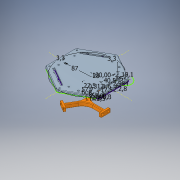
# Autodesk Inventor part: Stewart-Platform-Base-Innen
Saved by Autodesk Inventor 2018.2 (Build 222227000, 227)
## iProperties
Created: 2018-02-17
Part Number: Stewart-Platform-Base-Innen
Material: Generisch
Document SubType Name: Modeling
Designer: JochenAlt
Density: 1 g/cm^3
Appearance: Vorgabe
Author: JochenAlt
Autodesk Inventor part; units mm, degrees
ref_plane "YZ Plane" through (0, 0, 0) normal (1, 0, 0) x (0, 1, 0)
ref_plane "XZ Plane" through (0, 0, 0) normal (0, 1, 0) x (-1, 0, 0)
sketch "Skizze1" plane through (0, 0, 0) normal (0, 0, 1) x (1, 0, 0)
  line L0 (0, 78.1556) -> (0, -78.0893) construction
  line L1 (-71.7181, 0) -> (82.4088, 0) construction
  line L2 (31.6, 28.85) -> (44.1, 28.85) construction
  line L3 (47.4, 25.55) -> (47.4, -25.55) construction
  line L4 (44.1, -28.85) -> (31.6, -28.85) construction
  line L5 (28.3, -25.55) -> (28.3, 25.55) construction
  arc A0 (31.6, 28.85) -> (28.3, 25.55) centre (31.6, 25.55) ccw construction
  arc A1 (47.4, 25.55) -> (44.1, 28.85) centre (44.1, 25.55) ccw construction
  arc A2 (44.1, -28.85) -> (47.4, -25.55) centre (44.1, -25.55) ccw construction
  arc A3 (28.3, -25.55) -> (31.6, -28.85) centre (31.6, -25.55) ccw construction
  circle A4 centre (31.6, 25.55) radius 1.25
  circle A5 centre (44.1, 25.55) radius 1.25
  circle A6 centre (31.6, -25.55) radius 1.25
  circle A7 centre (44.1, -25.55) radius 1.25
  line L6 (41.4, 20.25) -> (41.4, -20.25)
  line L7 (38.3, 20.25) -> (38.3, -20.25)
  line L8 (38.3, 20.25) -> (41.4, 20.25)
  line L9 (38.3, -20.25) -> (41.4, -20.25)
  line L10 (38.3, 0.8) -> (41.4, 0.8)
  line L11 (38.3, -0.8) -> (41.4, -0.8)
  line L12 (41.4, 11.55) -> (44.416, 11.55)
  line L13 (44.416, 11.55) -> (44.416, 8.75)
  line L14 (44.416, 8.75) -> (41.4, 8.75)
  line L15 (41.4, -8.75) -> (44.416, -8.75)
  line L16 (44.416, -8.75) -> (44.416, -11.55)
  line L17 (44.416, -11.55) -> (41.4, -11.55)
  line L18 (44.1, 29.15) -> (31.6, 29.15)
  arc A8 (31.6, 29.15) -> (28, 25.55) centre (31.6, 25.55) ccw
  line L19 (28, 25.55) -> (28, -25.55)
  arc A9 (28, -25.55) -> (31.6, -29.15) centre (31.6, -25.55) ccw
  line L20 (31.6, -29.15) -> (44.1, -29.15)
  arc A10 (44.1, -29.15) -> (47.7, -25.55) centre (44.1, -25.55) ccw
  line L21 (47.7, -25.55) -> (47.7, 25.55)
  arc A11 (47.7, 25.55) -> (44.1, 29.15) centre (44.1, 25.55) ccw
  line L22 (26.117, -29.2238) -> (28.6093, -27.5539) construction
  line L23 (49.7, 0) -> (47.7, 0) construction
  circle A12 centre (0, 0) radius 49.7 construction
  line L24 (35.8007, 29.2532) -> (34.3005, 27.9307) construction
  line L25 (47.7, -19.95) -> (41.4, -19.95)
  line L26 (47.7, 19.95) -> (41.4, 19.95)
  arc A13 (3.1946, 52.7667) -> (-1.7231, 54.0844) centre (0.0769, 50.9667) ccw
  circle A14 centre (0.0769, 50.9667) radius 1.25
  line L27 (-1.7231, 54.0844) -> (-45.9769, 28.5344)
  line L28 (-6.5728, 51.2844) -> (-3.4228, 45.8285)
  line L29 (-12.2054, 44.2404) -> (-10.6974, 41.6285)
  line L30 (-14.6303, 42.8404) -> (-12.2054, 44.2404)
  line L31 (-13.1223, 40.2285) -> (-14.6303, 42.8404)
  line L32 (-38.237, 25.7285) -> (-3.163, 45.9785)
  line L33 (-1.613, 43.2938) -> (-3.163, 45.9785)
  line L34 (-36.687, 23.0438) -> (-1.613, 43.2938)
  line L35 (-18.4572, 33.5688) -> (-20.0072, 36.2535)
  line L36 (-19.8428, 32.7688) -> (-21.3928, 35.4535)
  line L37 (-32.2106, 32.6904) -> (-29.7857, 34.0904)
  line L38 (-29.7857, 34.0904) -> (-28.2777, 31.4785)
  line L39 (-30.7026, 30.0785) -> (-32.2106, 32.6904)
  line L40 (-41.1272, 31.3344) -> (-37.9772, 25.8785)
  line L41 (-36.687, 23.0438) -> (-38.237, 25.7285)
  arc A15 (-45.9769, 28.5344) -> (-47.2946, 23.6167) centre (-44.1769, 25.4167) ccw
  circle A16 centre (-44.1769, 25.4167) radius 1.25
  line L42 (-47.2946, 23.6167) -> (-41.0446, 12.7914)
  circle A17 centre (6.3269, 40.1414) radius 1.25
  arc A18 (8.1269, 37.0237) -> (9.4446, 41.9414) centre (6.3269, 40.1414) ccw
  line L43 (-36.1269, 11.4737) -> (8.1269, 37.0237)
  circle A19 centre (-37.9269, 14.5914) radius 1.25
  arc A20 (-41.0446, 12.7914) -> (-36.1269, 11.4737) centre (-37.9269, 14.5914) ccw
  line L44 (9.4446, 41.9414) -> (3.1946, 52.7667)
  arc A21 (-47.2946, -23.6167) -> (-45.9769, -28.5344) centre (-44.1769, -25.4167) ccw
  circle A22 centre (-44.1769, -25.4167) radius 1.25
  line L45 (-45.9769, -28.5344) -> (-1.7231, -54.0844)
  line L46 (-41.1272, -31.3344) -> (-37.9772, -25.8785)
  line L47 (-32.2106, -32.6904) -> (-30.7026, -30.0785)
  line L48 (-29.7857, -34.0904) -> (-32.2106, -32.6904)
  line L49 (-28.2777, -31.4785) -> (-29.7857, -34.0904)
  line L50 (-3.163, -45.9785) -> (-38.237, -25.7285)
  line L51 (-36.687, -23.0438) -> (-38.237, -25.7285)
  line L52 (-1.613, -43.2938) -> (-36.687, -23.0438)
  line L53 (-19.8428, -32.7688) -> (-21.3928, -35.4535)
  line L54 (-18.4572, -33.5688) -> (-20.0072, -36.2535)
  line L55 (-12.2054, -44.2404) -> (-14.6303, -42.8404)
  line L56 (-14.6303, -42.8404) -> (-13.1223, -40.2285)
  line L57 (-10.6974, -41.6285) -> (-12.2054, -44.2404)
  line L58 (-6.5728, -51.2844) -> (-3.4228, -45.8285)
  line L59 (-1.613, -43.2938) -> (-3.163, -45.9785)
  arc A23 (-1.7231, -54.0844) -> (3.1946, -52.7667) centre (0.0769, -50.9667) ccw
  circle A24 centre (0.0769, -50.9667) radius 1.25
  line L60 (3.1946, -52.7667) -> (9.4446, -41.9414)
  circle A25 centre (-37.9269, -14.5914) radius 1.25
  arc A26 (-36.1269, -11.4737) -> (-41.0446, -12.7914) centre (-37.9269, -14.5914) ccw
  line L61 (8.1269, -37.0237) -> (-36.1269, -11.4737)
  circle A27 centre (6.3269, -40.1414) radius 1.25
  arc A28 (9.4446, -41.9414) -> (8.1269, -37.0237) centre (6.3269, -40.1414) ccw
  line L62 (-41.0446, -12.7914) -> (-47.2946, -23.6167)
  line L63 (48.4856, -28.1531) -> (47.1957, -27.3875) construction
  line L64 (49.2, -25.55) -> (49.2, 25.55)
  line L65 (-2.3204, -55.1191) -> (-46.5743, -29.5691)
  line L66 (-46.6082, 29.6278) -> (-2.3543, 55.1778)
  arc A29 (-46.6082, 29.6278) -> (-49.0395, 25.4102) centre (-44.1769, 25.4167) ccw
  line L67 (2.4885, 55.1891) -> (46.6293, 29.9786)
  line L68 (-48.9717, -25.4231) -> (-49.0395, 25.4102)
  arc A30 (2.4885, 55.1891) -> (-2.3543, 55.1778) centre (0.0769, 50.9667) ccw
  arc A31 (49.2, 25.55) -> (46.6293, 29.9786) centre (44.1, 25.55) ccw
  arc A32 (32.9365, 29.15) -> (44.8907, 37.253) centre (44.1, 25.55) ccw
  arc A33 (46.6234, -29.982) -> (49.2, -25.55) centre (44.1, -25.55) ccw
  line L69 (46.6234, -29.982) -> (2.4494, -55.1334)
  arc A34 (-2.3204, -55.1191) -> (2.4494, -55.1334) centre (0.0769, -50.9667) ccw
  arc A35 (-48.9717, -25.4231) -> (-46.5743, -29.5691) centre (-44.1769, -25.4167) ccw
  circle A36 centre (0, 0) radius 43.5 construction
  circle A37 centre (-43.5, 0) radius 1.65
  circle A38 centre (21.75, -37.6721) radius 1.65
  circle A39 centre (21.75, 37.6721) radius 1.65
  line L70 (21.75, -37.6721) -> (0, 0) construction
  line L71 (0, 0) -> (21.75, 37.6721) construction
  line L72 (34.4282, 0) -> (34.4282, -12) construction
  line L73 (34.4282, -12) -> (6.9282, -12) construction
  point P0 (44.416, -10.15)
  point P1 (0, 0)
  point P2 (47.7, -21.4)
  point P3 (47.7, 21.4)
  point P4 (-23.85, 41.3094)
  point P5 (-5.3171, 52.0094)
  point P6 (-42.3829, 30.6094)
  point P7 (-13.4178, 43.5404)
  point P8 (9.5577, 38.5533)
  point P9 (-41.3389, 15.7397)
  point P10 (-23.85, -41.3094)
  point P11 (-42.3829, -30.6094)
  point P12 (-5.3171, -52.0094)
  point P13 (-30.9982, -33.3904)
  point P14 (-38.167, -10.9994)
  point P15 (7.0384, -43.6704)
  dimension "d1" = 57.7
  dimension "d2" = 19.1
  dimension "d3" = 3.3
  dimension "d5" = 2.5
  dimension "d6" = 6
  dimension "d7" = 3.1
  dimension "d9" = 1.6
  dimension "d10" = 2.984
  dimension "d11" = 2.8
  dimension "d12" = 17.5
  dimension "d21" = 0.3
  dimension "d22" = 3
  dimension "d34" = 2
  dimension "d35" = 2
  dimension "d105" = 360
  dimension "d107" = 40.5
  dimension "d108" = 0.3
  dimension "d140" = 1.5
  dimension "d141" = 28
  dimension "d145" = 1.5
  dimension "d148" = 87
  dimension "d149" = 3.3
  dimension "d150" = 120
  dimension "d151" = 12
  dimension "d152" = 27.5
  constraints: 138 end point, 56 point on circle, 39 centre point, 28 point on line, 22 coincident, 20 tangent, 11 horizontal, 8 equal radius, 7 parallel, 5 perpendicular, 3 line through centre, 2 midpoint, 2 vertical, 1 collinear, 1 horizontal alignment, 1 symmetric about line, 253 other
  measures "d1" distance between parallel lines of L4 L2
  measures "d2" distance between parallel lines of L3 L5
  measures "d3" radius of A0
  measures "d5" diameter of A4
  measures "d9" distance between parallel lines of L11 L10
  measures "d10" distance between parallel lines of L3 L13
  measures "d11" distance between parallel lines of L14 L12
  measures "d12" distance between parallel lines of L15 L14
  measures "d21" distance between parallel lines of L19 L5
  measures "d22" distance of L22.end L22.start
  measures "d34" distance of L23.start L23.end
  measures "d35" distance of L24.start L24.end
  measures "d107" distance between parallel lines of L8 L9
  measures "d108" distance between parallel lines of L25 L9
  measures "d140" distance of L63.start L63.end
  measures "d141" distance between parallel lines of L0 L19
  measures "d145" distance between parallel lines of L21 L64
  measures "d148" diameter of A36
  measures "d149" diameter of A37
  measures "d150" angle of L71 L70
  measures "d151" distance of L72.start L72.end
  measures "d152" distance of L72.end L73.end
extrude "Extrusion5" add sketch "Skizze1" along normal blind 4 contours A4 A32 L18 A11 L21 L26 L6 L8 L7 | A4 A32 L7 L9 L6 L25 L21 A10 L20 A9 L19 A8 L18 | A32 L21 L25 L6 L17 L16 L15 L14 L13 L12 | L6 L26 L21 A32 | L44 A18 L43 A20 L42 A15 L27 L40 L32 L41 L34 L33 L28 A13 | L28 L32 L29 L30 L31 L38 L37 L39 L40 L27 | L62 A26 L61 A28 L60 A23 L45 L58 L50 L59 L52 L51 L46 A21 | L46 L50 L47 L48 L49 L56 L55 L57 L58 L45 | A33 L69 A34 L65 A35 L68 A29 L66 A30 L67 A31 L64
extrude "Extrusion4" cut sketch "Skizze1" along normal blind 2 contours A4 A32 L18 A11 L21 L26 L6 L8 L7 | A4 A32 L7 L9 L6 L25 L21 A10 L20 A9 L19 A8 L18 | L12 L13 L14 L6 | L15 L16 L17 L6 | L44 A18 L43 A20 L42 A15 L27 L40 L32 L41 L34 L33 L28 A13 | L62 A26 L61 A28 L60 A23 L45 L58 L50 L59 L52 L51 L46 A21
ref_plane "Arbeitsebene2" through (0, 0, -40.8) normal (0, 0, 1) x (1, 0, 0)
sketch "Skizze6" plane through (0, 0, -40.8) normal (0, 0, 1) x (1, 0, 0)
  line L0 (41.4, -11.55) -> (41.4, -20.25) construction
  line L1 (41.4, -20.25) -> (38.3, -20.25) construction
  line L2 (38.3, -20.25) -> (38.3, 20.25) construction
  line L3 (41.4, 20.25) -> (41.4, 11.55) construction
  line L4 (38.3, 20.25) -> (41.4, 20.25) construction
  circle A0 centre (44.1, -25.55) radius 1.25 construction
  circle A1 centre (31.6, -25.55) radius 1.25 construction
  circle A2 centre (44.1, 25.55) radius 1.25 construction
  circle A3 centre (31.6, 25.55) radius 1.25 construction
  line L5 (34.1, 8.75) -> (34.1, -8.75)
  line L6 (34.1, 8.75) -> (31.1, 8.75)
  line L7 (41.4, -8.75) -> (41.4, 8.75) projected
  line L8 (-65.8313, 0) -> (60.3802, 0) construction
  line L9 (0, 37.52) -> (0, -37.52) construction
  line L10 (31.1, -8.75) -> (31.1, -2)
  line L11 (31.1, 2) -> (31.1, 8.75)
  line L12 (0, 0) -> (8.9019, 15.4186) construction
  line L13 (0, 0) -> (9.1171, -15.7912) construction
  arc A4 (2.7017, 4.6795) -> (12.7017, 2) centre (12.7017, 22) ccw
  arc A5 (12.7017, -2) -> (2.7017, -4.6795) centre (12.7017, -22) ccw
  line L14 (2.7017, 4.6795) -> (0, 6.2393)
  line L15 (2.7017, -4.6795) -> (0, -6.2393)
  line L16 (31.1, 2) -> (12.7017, 2)
  line L17 (31.1, -2) -> (12.7017, -2)
  line L18 (31.1, 8.75) -> (34.1, 8.75) projected
  line L19 (34.1, -8.75) -> (31.1, -8.75)
  arc A6 (0, -1.65) -> (0, 1.65) centre (0, 0) ccw
  line L20 (0, 6.2393) -> (0, 1.65)
  line L21 (0, -1.65) -> (0, -6.2393)
  line L22 (41.4, 8.75) -> (41.4, -8.75) projected
  line L23 (41.4, -8.75) -> (44.416, -8.75) projected
  line L24 (44.416, -8.75) -> (44.416, -11.55) projected
  line L25 (44.416, -11.55) -> (41.4, -11.55) projected
  line L26 (41.4, 11.55) -> (44.416, 11.55) projected
  line L27 (44.416, 11.55) -> (44.416, 8.75) projected
  line L28 (44.416, 8.75) -> (41.4, 8.75) projected
  point P0 (-47.8011, -0.8)
  dimension "d73" = 120
  dimension "d89" = 20
  dimension "d90" = 4
  dimension "d91" = 3.3
  dimension "d146" = 3
  dimension "d147" = 4.2
  constraints: 26 end point, 6 point on circle, 4 perpendicular, 4 point on line, 4 tangent, 3 centre point, 2 parallel, 1 coincident, 1 collinear, 1 other
  measures "d73" angle of L13 L12
  measures "d89" radius of A5
  measures "d90" distance between parallel lines of L16 L17
  measures "d91" diameter of A6
  measures "d146" distance between parallel lines of L11 L5
  measures "d147" distance between parallel lines of L5 L2
extrude "Extrusion9" add sketch "Skizze6" against normal blind 7.1 separate body
sketch "Skizze7" plane through (34.1, 8.75, -40.8) normal (1, 0, 0) x (0, 0, -1)
  circle A0 centre (3.8, -3.7) radius 1.7
  circle A1 centre (3.8, -13.8) radius 1.7
  line L0 (0, -17.5) -> (0, 0) construction
  line L1 (0, -8.75) -> (7.1, -8.75) construction
  line L2 (7.1, 0) -> (7.1, -17.5) construction
  point P0 (-40.8, -8.75)
  dimension "d76" = 3.4
  dimension "d77" = 10.1
  dimension "d88" = 3.3
  constraints: 2 centre point, 2 end point, 2 midpoint, 1 equal radius, 1 symmetric about line
  measures "d76" diameter of A1
  measures "d77" distance of A0.centre A1.centre
  measures "d88" distance from line of A0.centre L2
extrude "Extrusion10" cut sketch "Skizze7" against normal blind 10 bodies 1 2
pattern_circular "Runde Anordnung5" count 3 over 360 about axis through (0, 0, -10) along (0, 0, 1) of "Extrusion10", "Extrusion9" bodies 2
fillet "Rundung1" radius 1 30 edges at (2.7017, 4.6795, -40.8) (21.9009, 2, -40.8) (-9.2184, 19.9667, -40.8) (2.7017, -4.6795, -40.8) (-9.2184, -19.9667, -40.8) (21.9009, -2, -40.8) (-12.6825, -17.9667, -40.8) (-12.6825, 17.9667, -40.8) (-5.4034, 0, -40.8) (2.7017, 4.6795, -47.9) (21.9009, 2, -47.9) (-9.2184, 19.9667, -47.9) (-12.6825, 17.9667, -47.9) (-12.6825, -17.9667, -47.9) (-5.4034, 0, -47.9) (32.6, -8.75, -47.9) (32.6, 8.75, -47.9) (-8.7223, -32.6074, -47.9) (-23.8777, -23.8574, -47.9) (-23.8777, -23.8574, -40.8) (-8.7223, -32.6074, -40.8) (32.6, -8.75, -40.8) (32.6, 8.75, -40.8) (-8.7223, 32.6074, -40.8) (-8.7223, 32.6074, -47.9) (-23.8777, 23.8574, -40.8) (-23.8777, 23.8574, -47.9) (-9.2184, -19.9667, -47.9) (21.9009, -2, -47.9) (2.7017, -4.6795, -47.9)
fillet "Rundung2" radius 1 15 edges at (-24.4474, -42.3441, 4) (49.2, 0, 4) (-24.4813, 42.4028, 4) (48.5091, -28.1132, 0) (49.2, 0, 0) (48.5108, 28.1103, 0) (24.5589, 42.5838, 0) (0.0656, 55.8292, 0) (-24.4813, 42.4028, 0) (-48.3896, 27.8452, 0) (-49.0056, -0.0064, 0) (-48.3278, -27.8169, 0) (-24.4474, -42.3441, 0) (0.0626, -55.7615, 0) (24.5364, -42.5577, 0)
sketch "Skizze8" plane through (0, 0, 4) normal (0, 0, 1) x (1, 0, 0)
  circle A0 centre (6.3269, -40.1414) radius 1.25 construction
  circle A1 centre (-37.9269, -14.5914) radius 1.25 construction
  circle A2 centre (0.0769, -50.9667) radius 1.25 construction
  circle A3 centre (-44.1769, -25.4167) radius 1.25 construction
  circle A4 centre (-37.9269, 14.5914) radius 1.25 construction
  circle A5 centre (6.3269, 40.1414) radius 1.25 construction
  circle A6 centre (-44.1769, 25.4167) radius 1.25 construction
  circle A7 centre (0.0769, 50.9667) radius 1.25 construction
  circle A8 centre (44.1, -25.55) radius 1.25 construction
  circle A9 centre (31.6, -25.55) radius 1.25 construction
  circle A10 centre (44.1, 25.55) radius 1.25 construction
  circle A11 centre (31.6, 25.55) radius 1.25 construction
  line L0 (-13.1223, -40.2285) -> (-28.2777, -31.4785) construction
  line L1 (-30.7026, -30.0785) -> (-38.237, -25.7285) construction
  line L2 (-38.237, -25.7285) -> (-36.687, -23.0438) construction
  line L3 (-36.687, -23.0438) -> (-1.613, -43.2938) construction
  line L4 (-1.613, -43.2938) -> (-3.163, -45.9785) construction
  line L5 (-28.2777, 31.4785) -> (-13.1223, 40.2285) construction
  line L6 (-10.6974, 41.6285) -> (-3.163, 45.9785) construction
  line L7 (-3.163, 45.9785) -> (-1.613, 43.2938) construction
  line L8 (-1.613, 43.2938) -> (-36.687, 23.0438) construction
  line L9 (-36.687, 23.0438) -> (-38.237, 25.7285) construction
  line L10 (41.4, 20.25) -> (41.4, 11.55) construction
  line L11 (38.3, -20.25) -> (38.3, 20.25) construction
  line L12 (38.3, 20.25) -> (41.4, 20.25) construction
  line L13 (41.4, -11.55) -> (41.4, -20.25) construction
  line L14 (41.4, -20.25) -> (38.3, -20.25) construction
  line L15 (41.4, -11.55) -> (44.416, -11.55) projected
  line L16 (41.4, 8.75) -> (44.416, 8.75) projected
  line L17 (44.416, 11.55) -> (41.4, 11.55) projected
  line L18 (42.216, 8.75) -> (44.416, 8.75)
  line L19 (44.416, 8.75) -> (44.416, 11.55)
  line L20 (44.416, 11.55) -> (42.216, 11.55)
  line L21 (42.216, 11.55) -> (42.216, 8.75)
  line L22 (-29.7857, -34.0904) -> (-28.2777, -31.4785) projected
  line L23 (-28.6857, -32.1851) -> (-13.5303, -40.9351) construction
  line L24 (-28.6857, 32.1851) -> (-13.5303, 40.9351) construction
  line L25 (-13.1223, 40.2285) -> (-14.6303, 42.8404) construction
  line L26 (-29.7857, 34.0904) -> (-28.2777, 31.4785) projected
  line L27 (-28.6857, 32.1851) -> (-29.7857, 34.0904)
  line L28 (-29.7857, 34.0904) -> (-32.2106, 32.6904)
  line L29 (-32.2106, 32.6904) -> (-31.1106, 30.7851)
  line L30 (-31.1106, 30.7851) -> (-28.6857, 32.1851)
  line L31 (-13.5303, 40.9351) -> (-14.6303, 42.8404)
  line L32 (-14.6303, 42.8404) -> (-12.2054, 44.2404)
  line L33 (-12.2054, 44.2404) -> (-11.1054, 42.3351)
  line L34 (-11.1054, 42.3351) -> (-13.5303, 40.9351)
  line L35 (-13.5303, -40.9351) -> (-14.6303, -42.8404)
  line L36 (-14.6303, -42.8404) -> (-12.2054, -44.2404)
  line L37 (-12.2054, -44.2404) -> (-11.1054, -42.3351)
  line L38 (-11.1054, -42.3351) -> (-13.5303, -40.9351)
  line L39 (-28.6857, -32.1851) -> (-29.7857, -34.0904)
  line L40 (-29.7857, -34.0904) -> (-32.2106, -32.6904)
  line L41 (-32.2106, -32.6904) -> (-31.1106, -30.7851)
  line L42 (-31.1106, -30.7851) -> (-28.6857, -32.1851)
  line L43 (-13.1223, 40.2285) -> (-14.6303, 42.8404) projected
  line L44 (-14.6303, 42.8404) -> (-12.2054, 44.2404) projected
  line L45 (-12.2054, 44.2404) -> (-10.6974, 41.6285) projected
  line L46 (-38.237, 25.7285) -> (-30.7026, 30.0785) projected
  line L47 (-30.7026, 30.0785) -> (-32.2106, 32.6904) projected
  line L48 (-32.2106, 32.6904) -> (-29.7857, 34.0904) projected
  line L49 (-29.7857, 34.0904) -> (-28.2777, 31.4785) projected
  line L50 (41.4, 8.75) -> (41.4, -8.75) projected
  line L51 (41.4, -8.75) -> (44.416, -8.75) projected
  line L52 (44.416, -8.75) -> (44.416, -11.55) projected
  line L53 (44.416, -11.55) -> (41.4, -11.55) projected
  line L54 (41.4, 11.55) -> (44.416, 11.55) projected
  line L55 (44.416, 11.55) -> (44.416, 8.75) projected
  line L56 (44.416, 8.75) -> (41.4, 8.75) projected
  line L57 (-3.163, -45.9785) -> (-10.6974, -41.6285) projected
  line L58 (-10.6974, -41.6285) -> (-12.2054, -44.2404) projected
  line L59 (-12.2054, -44.2404) -> (-14.6303, -42.8404) projected
  line L60 (-14.6303, -42.8404) -> (-13.1223, -40.2285) projected
  line L61 (-28.2777, -31.4785) -> (-29.7857, -34.0904) projected
  line L62 (-29.7857, -34.0904) -> (-32.2106, -32.6904) projected
  line L63 (-32.2106, -32.6904) -> (-30.7026, -30.0785) projected
  arc A12 (44.1, -29.15) -> (47.7, -25.55) centre (44.1, -25.55) ccw construction
  line L64 (47.7, -19.95) -> (41.4, -19.95) construction
  line L65 (41.4, -19.95) -> (41.4, -11.55) construction
  line L66 (41.4, -11.55) -> (44.416, -11.55) construction
  line L67 (44.416, -11.55) -> (44.416, -8.75) construction
  line L68 (44.416, -8.75) -> (41.4, -8.75) construction
  line L69 (41.4, -8.75) -> (41.4, 8.75) construction
  line L70 (41.4, 8.75) -> (44.416, 8.75) construction
  line L71 (44.416, 8.75) -> (44.416, 11.55) construction
  line L72 (44.416, 11.55) -> (41.4, 11.55) construction
  line L73 (41.4, 11.55) -> (41.4, 19.95) construction
  line L74 (41.4, 19.95) -> (47.7, 19.95) construction
  arc A13 (47.7, 25.55) -> (44.1, 29.15) centre (44.1, 25.55) ccw construction
  circle A14 centre (44.1, -25.55) radius 1.25 construction
  circle A15 centre (31.6, -25.55) radius 1.25 construction
  circle A16 centre (44.1, 25.55) radius 1.25 construction
  circle A17 centre (31.6, 25.55) radius 1.25 construction
  line L75 (41.4, 20.25) -> (41.4, 19.95) construction
  line L76 (38.3, 20.25) -> (41.4, 20.25) construction
  line L77 (38.3, -20.25) -> (38.3, 20.25) construction
  line L78 (41.4, -20.25) -> (38.3, -20.25) construction
  line L79 (41.4, -19.95) -> (41.4, -20.25) construction
  line L80 (47.7, -19.95) -> (41.4, -19.95) construction
  line L81 (47.7, -25.55) -> (47.7, -19.95) construction
  arc A18 (44.1, -29.15) -> (47.7, -25.55) centre (44.1, -25.55) ccw construction
  line L82 (31.6, -29.15) -> (44.1, -29.15) construction
  arc A19 (28, -25.55) -> (31.6, -29.15) centre (31.6, -25.55) ccw construction
  line L83 (28, 25.55) -> (28, -25.55) construction
  arc A20 (31.6, 29.15) -> (28, 25.55) centre (31.6, 25.55) ccw construction
  line L84 (44.1, 29.15) -> (31.6, 29.15) construction
  arc A21 (47.7, 25.55) -> (44.1, 29.15) centre (44.1, 25.55) ccw construction
  line L85 (47.7, 19.95) -> (47.7, 25.55) construction
  line L86 (41.4, 19.95) -> (47.7, 19.95) construction
  line L87 (44.416, -8.75) -> (41.4, -8.75) projected
  line L88 (44.416, -8.75) -> (42.216, -8.75)
  line L89 (42.216, -8.75) -> (42.216, -11.55)
  line L90 (42.216, -11.55) -> (44.416, -11.55)
  line L91 (44.416, -11.55) -> (44.416, -8.75)
  line L92 (42.216, 8.75) -> (42.216, -8.75) construction
  line L93 (41.4, -8.75) -> (44.416, -8.75) construction
  line L94 (47.7, 19.95) -> (47.7, 25.55) projected
  line L95 (44.1, 29.15) -> (31.6, 29.15) projected
  arc A22 (31.6, 29.15) -> (28, 25.55) centre (31.6, 25.55) ccw projected
  line L96 (28, 25.55) -> (28, -25.55) projected
  arc A23 (28, -25.55) -> (31.6, -29.15) centre (31.6, -25.55) ccw projected
  line L97 (31.6, -29.15) -> (44.1, -29.15) projected
  line L98 (47.7, -25.55) -> (47.7, -19.95) projected
  arc A24 (-41.0446, 12.7914) -> (-36.1269, 11.4737) centre (-37.9269, 14.5914) ccw projected
  arc A25 (-36.1269, -11.4737) -> (-41.0446, -12.7914) centre (-37.9269, -14.5914) ccw projected
  line L99 (8.1269, -37.0237) -> (-36.1269, -11.4737) projected
  arc A26 (9.4446, -41.9414) -> (8.1269, -37.0237) centre (6.3269, -40.1414) ccw projected
  arc A27 (8.1269, 37.0237) -> (9.4446, 41.9414) centre (6.3269, 40.1414) ccw projected
  line L100 (-36.1269, 11.4737) -> (8.1269, 37.0237) projected
  line L101 (-47.2946, 23.6167) -> (-41.0446, 12.7914) projected
  arc A28 (-45.9769, 28.5344) -> (-47.2946, 23.6167) centre (-44.1769, 25.4167) ccw projected
  line L102 (-41.1272, 31.3344) -> (-45.9769, 28.5344) projected
  line L103 (-37.9772, 25.8785) -> (-41.1272, 31.3344) projected
  line L104 (-38.237, 25.7285) -> (-37.9772, 25.8785) projected
  line L105 (-36.687, 23.0438) -> (-38.237, 25.7285) projected
  line L106 (-1.613, 43.2938) -> (-36.687, 23.0438) projected
  line L107 (-3.163, 45.9785) -> (-1.613, 43.2938) projected
  line L108 (-3.4228, 45.8285) -> (-3.163, 45.9785) projected
  line L109 (-6.5728, 51.2844) -> (-3.4228, 45.8285) projected
  line L110 (-1.7231, 54.0844) -> (-6.5728, 51.2844) projected
  arc A29 (3.1946, 52.7667) -> (-1.7231, 54.0844) centre (0.0769, 50.9667) ccw projected
  line L111 (9.4446, 41.9414) -> (3.1946, 52.7667) projected
  line L112 (3.1946, -52.7667) -> (9.4446, -41.9414) projected
  arc A30 (-1.7231, -54.0844) -> (3.1946, -52.7667) centre (0.0769, -50.9667) ccw projected
  line L113 (-6.5728, -51.2844) -> (-1.7231, -54.0844) projected
  line L114 (-3.4228, -45.8285) -> (-6.5728, -51.2844) projected
  line L115 (-3.163, -45.9785) -> (-3.4228, -45.8285) projected
  line L116 (-1.613, -43.2938) -> (-3.163, -45.9785) projected
  line L117 (-36.687, -23.0438) -> (-1.613, -43.2938) projected
  line L118 (-38.237, -25.7285) -> (-36.687, -23.0438) projected
  line L119 (-37.9772, -25.8785) -> (-38.237, -25.7285) projected
  line L120 (-41.1272, -31.3344) -> (-37.9772, -25.8785) projected
  line L121 (-45.9769, -28.5344) -> (-41.1272, -31.3344) projected
  arc A31 (-47.2946, -23.6167) -> (-45.9769, -28.5344) centre (-44.1769, -25.4167) ccw projected
  line L122 (-41.0446, -12.7914) -> (-47.2946, -23.6167) projected
  arc A32 (8.1269, 37.0237) -> (9.4446, 41.9414) centre (6.3269, 40.1414) ccw projected
  arc A33 (9.4446, -41.9414) -> (8.1269, -37.0237) centre (6.3269, -40.1414) ccw projected
  line L123 (8.1269, -37.0237) -> (-36.1269, -11.4737) projected
  arc A34 (-36.1269, -11.4737) -> (-41.0446, -12.7914) centre (-37.9269, -14.5914) ccw projected
  arc A35 (-41.0446, 12.7914) -> (-36.1269, 11.4737) centre (-37.9269, 14.5914) ccw projected
  line L124 (-36.1269, 11.4737) -> (8.1269, 37.0237) projected
  line L125 (-41.1272, -31.3344) -> (-37.9772, -25.8785) projected
  line L126 (-37.9772, -25.8785) -> (-30.7026, -30.0785) projected
  line L127 (-30.7026, -30.0785) -> (-32.2106, -32.6904) projected
  line L128 (-32.2106, -32.6904) -> (-29.7857, -34.0904) projected
  line L129 (-29.7857, -34.0904) -> (-28.2777, -31.4785) projected
  line L130 (-28.2777, -31.4785) -> (-13.1223, -40.2285) projected
  line L131 (-13.1223, -40.2285) -> (-14.6303, -42.8404) projected
  line L132 (-14.6303, -42.8404) -> (-12.2054, -44.2404) projected
  line L133 (-12.2054, -44.2404) -> (-10.6974, -41.6285) projected
  line L134 (-10.6974, -41.6285) -> (-3.4228, -45.8285) projected
  line L135 (-3.4228, -45.8285) -> (-6.5728, -51.2844) projected
  line L136 (-6.5728, -51.2844) -> (-1.7231, -54.0844) projected
  arc A36 (-1.7231, -54.0844) -> (3.1946, -52.7667) centre (0.0769, -50.9667) ccw projected
  line L137 (3.1946, -52.7667) -> (9.4446, -41.9414) projected
  line L138 (9.4446, 41.9414) -> (3.1946, 52.7667) projected
  arc A37 (3.1946, 52.7667) -> (-1.7231, 54.0844) centre (0.0769, 50.9667) ccw projected
  line L139 (-1.7231, 54.0844) -> (-6.5728, 51.2844) projected
  line L140 (-6.5728, 51.2844) -> (-3.4228, 45.8285) projected
  line L141 (-3.4228, 45.8285) -> (-10.6974, 41.6285) projected
  line L142 (-10.6974, 41.6285) -> (-12.2054, 44.2404) projected
  line L143 (-12.2054, 44.2404) -> (-14.6303, 42.8404) projected
  line L144 (-14.6303, 42.8404) -> (-13.1223, 40.2285) projected
  line L145 (-13.1223, 40.2285) -> (-28.2777, 31.4785) projected
  line L146 (-28.2777, 31.4785) -> (-29.7857, 34.0904) projected
  line L147 (-29.7857, 34.0904) -> (-32.2106, 32.6904) projected
  line L148 (-32.2106, 32.6904) -> (-30.7026, 30.0785) projected
  line L149 (-30.7026, 30.0785) -> (-37.9772, 25.8785) projected
  line L150 (-37.9772, 25.8785) -> (-41.1272, 31.3344) projected
  line L151 (-41.1272, 31.3344) -> (-45.9769, 28.5344) projected
  arc A38 (-45.9769, 28.5344) -> (-47.2946, 23.6167) centre (-44.1769, 25.4167) ccw projected
  line L152 (-47.2946, 23.6167) -> (-41.0446, 12.7914) projected
  line L153 (-41.0446, -12.7914) -> (-47.2946, -23.6167) projected
  arc A39 (-47.2946, -23.6167) -> (-45.9769, -28.5344) centre (-44.1769, -25.4167) ccw projected
  line L154 (-45.9769, -28.5344) -> (-41.1272, -31.3344) projected
  point P0 (0, 0)
  dimension "d142" = 0.816
  dimension "d144" = 0.816
  constraints: 54 end point, 13 parallel, 7 perpendicular, 4 point on line, 2 collinear, 1 horizontal
  measures "d142" distance between parallel lines of L5 L24
  measures "d144" distance between parallel lines of L50 L92
extrude "Extrusion11" add sketch "Skizze8" against normal blind 4 contours L89 L51 L52 L15 | L21 L17 L19 L16 | L40 L41 L42 L22 | L38 L37 L36 L35 | L26 L30 L29 L28 | L31 L32 L33 L34 bodies 1
chamfer "Fase3" distance 2 distance2 4 1 edges at (-12.3178, -41.6351, 0) measured on face at (-12.5678, -42.0681, 0)
chamfer "Fase4" distance 2 distance2 4 1 edges at (-29.8982, -31.4851, 0) measured on face at (-30.1482, -31.9181, 0)
chamfer "Fase5" distance 2 distance2 4 1 edges at (-12.3178, 41.6351, 0) measured on face at (-12.5678, 42.0681, 0)
chamfer "Fase6" distance 2 distance2 4 1 edges at (-29.8982, 31.4851, 0) measured on face at (-30.1482, 31.9181, 0)
chamfer "Fase7" distance 2 distance2 4 1 edges at (42.216, -10.15, 0) measured on face at (42.716, -10.15, 0)
chamfer "Fase8" distance 2 distance2 4 1 edges at (42.216, 10.15, 0) measured on face at (42.716, 10.15, 0)
equation "\"d22\" = d20"
equation "\"d35\" = d34"
equation "\"d44\" = d21"
equation "\"d20\" = 3"
